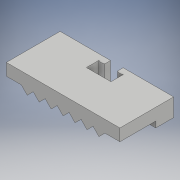
# Autodesk Inventor part: Clamp-part2(moving)-Base9x19mm.
Saved by Autodesk Inventor 2017 (Build 210142000, 142)
## iProperties
Created: 2021-08-04
Part Number: Clamp-part2(moving)-Base9x19mm.
Material: Generic
Document SubType Name: Modeling
Designer: Nikita
Density: 1 g/cm^3
Appearance: Default
Author: Nikita
Autodesk Inventor part; units mm, degrees
ref_plane "YZ Plane" through (0, 0, 0) normal (1, 0, 0) x (0, 1, 0)
ref_plane "XZ Plane" through (0, 0, 0) normal (0, 1, 0) x (-1, 0, 0)
ref_plane "XY Plane" through (0, 0, 0) normal (0, 0, 1) x (1, 0, 0)
sketch "Sketch1" plane through (0, 0, 0) normal (0, 0, 1) x (1, 0, 0)
  line L0 (0, 0) -> (19, 0)
  line L1 (19, 0) -> (19, 9)
  line L2 (19, 9) -> (0, 9)
  line L3 (0, 9) -> (0, 0)
  point P0 (9.5, 9)
  dimension "d0" = 19
  dimension "d1" = 9
  constraints: 8 end point, 2 parallel, 1 horizontal, 1 midpoint, 1 perpendicular
  measures "d0" distance of L2.end L1.end
  measures "d1" distance of L1.end L0.end
extrude "Extrusion1" add sketch "Sketch1" along normal blind 3
sketch "Sketch10" plane through (0, 0, 0) normal (-1, 0, 0) x (0, 0, 1)
  line L0 (0, 0) -> (3, 0) projected
  line L1 (3, 9) -> (3, 0) projected
  line L2 (3, 0) -> (2, 0)
  line L3 (2, 0) -> (2, 6)
  line L4 (2, 6) -> (3, 6)
  line L5 (3, 6) -> (3, 0)
  line L6 (3, 0) -> (2, 1)
  line L7 (3, 0) -> (4.4142, 0) construction
  line L8 (2, 1) -> (3, 2)
  line L9 (3, 0) -> (3, 9) projected
  line L10 (3, 2) -> (2, 3)
  line L11 (2, 3) -> (3, 4)
  line L12 (2, 5) -> (3, 4)
  line L13 (2, 5) -> (3, 5)
  dimension "d23" = 1
  dimension "d24" = 6
  dimension "d25" = 135
  dimension "d26" = 90
  constraints: 22 end point, 5 point on line, 3 perpendicular, 2 horizontal, 2 parallel, 1 equal length, 1 midpoint
  measures "d23" distance of L4.end L3.end
  measures "d24" distance of L2.end L3.end
  measures "d25" angle of L7 L6
  measures "d26" angle of L6 L8
extrude "Extrusion8" cut sketch "Sketch10" against normal up to next contours L6 L8 L1 | L10 L11 L1 | L12 L13 L1 | L3 L4 L1 L13
sketch "Sketch12" plane through (0, 0, 3) normal (0, 0, 1) x (1, 0, 0)
  line L0 (19, 9) -> (0, 9) projected
  line L1 (11.5494, 5.95) -> (7.4494, 5.95)
  line L2 (7.4494, 5.95) -> (7.4494, 8.05)
  line L3 (7.4494, 8.05) -> (11.5494, 8.05)
  line L4 (11.5494, 8.05) -> (11.5494, 5.95)
  line L5 (11.5494, 5.95) -> (7.4494, 8.05) construction
  line L6 (7.4494, 5.95) -> (11.5494, 8.05) construction
  line L7 (10.5494, 7.1) -> (8.4494, 7.1)
  line L8 (8.4494, 7.1) -> (8.4494, 9)
  line L9 (8.4494, 9) -> (10.5494, 9)
  line L10 (10.5494, 9) -> (10.5494, 7.1)
  line L11 (10.5494, 7.1) -> (8.4494, 9) construction
  line L12 (8.4494, 7.1) -> (10.5494, 9) construction
  point P0 (0, 0)
  point P1 (9.4994, 7)
  point P2 (9.4994, 8.05)
  dimension "d47" = 2
  dimension "d48" = 4.1
  dimension "d49" = 2.1
  dimension "d50" = 2.1
  constraints: 24 end point, 5 midpoint, 4 parallel, 2 horizontal, 2 perpendicular, 1 point on line
  measures "d47" distance from line of L0 point (9.499, 7)
  measures "d48" distance of L2.end L3.end
  measures "d49" distance of L1.end L2.end
  measures "d50" distance of L8.end L9.end
extrude "Extrusion10" cut sketch "Sketch12" against normal up to next
sketch "Sketch14" plane through (0, 0, 2) normal (0, 0, 1) x (1, 0, 0)
  line L0 (6.4994, 5) -> (12.4994, 5)
  line L1 (12.4994, 5) -> (12.4994, 6)
  line L2 (12.4994, 6) -> (6.4994, 6)
  line L3 (6.4994, 6) -> (6.4994, 5)
  line L4 (6.4994, 5) -> (12.4994, 6) construction
  line L5 (12.4994, 5) -> (6.4994, 6) construction
  line L6 (19, 9) -> (10.5494, 9) projected
  point P0 (0, 0)
  point P1 (9.4994, 5.5)
  dimension "d57" = 6
  dimension "d58" = 1
  dimension "d59" = 3.5
  constraints: 12 end point, 2 midpoint, 2 parallel, 1 horizontal, 1 perpendicular
  measures "d57" distance of L2.end L1.end
  measures "d58" distance of L1.end L0.end
  measures "d59" distance from line of L6 point (9.499, 5.5)
extrude "Extrusion12" add sketch "Sketch14" along normal blind 1
chamfer "Chamfer1" distance 0.5 angle 45 1 edges at (9.4994, 5, 3)
sketch "Sketch16" plane through (0, 0, 0) normal (0, 0, -1) x (-1, 0, 0)
  line L0 (-11.5494, 8.05) -> (-11.5494, 6) projected
  line L1 (-10.5494, 8.05) -> (-11.5494, 8.05) projected
  arc A0 (-11.5494, 8.05) -> (-10.5494, 8.05) centre (-11.0494, 8.916) ccw
  line L2 (-8.4494, 8.05) -> (-7.4494, 8.05) projected
  arc A1 (-8.4494, 8.05) -> (-7.4494, 8.05) centre (-7.9494, 8.916) ccw
  point P0 (0, 0)
  dimension "d66" = 1
  dimension "d67" = 1
  constraints: 4 point on circle, 2 centre point
  measures "d66" radius of A0
  measures "d67" radius of A1
extrude "Extrusion13" add sketch "Sketch16" against normal up to surface (3 mm away)
sketch "Sketch18" plane through (0, 0, 0) normal (0, -1, 0) x (1, 0, 0)
  line L0 (9.5, 3) -> (8.5, 2)
  line L1 (9.5, 3) -> (10.9142, 3) construction
  line L2 (8.5, 2) -> (7.5, 3)
  line L3 (7.5, 3) -> (6.4994, 2)
  line L4 (6.4994, 2) -> (5.5, 3)
  line L5 (5.5, 3) -> (4.5, 2)
  line L6 (5.5, 3) -> (6.9142, 3) construction
  line L7 (4.5, 2) -> (3.5, 3)
  line L8 (3.5, 3) -> (2.5, 2)
  line L9 (0, 3) -> (6.4994, 3) projected
  line L10 (0, 3) -> (3.5, 3)
  line L11 (19, 3) -> (19, 2)
  line L12 (19, 2) -> (16.5, 2)
  line L13 (0, 2) -> (0, 3)
  line L14 (8.5, 2) -> (6.4994, 2)
  line L15 (6.4994, 2) -> (4.5, 2)
  line L16 (4.5, 2) -> (2.5, 2)
  line L17 (3.5, 3) -> (5.5, 3)
  line L18 (5.5, 3) -> (7.5, 3)
  line L19 (7.5, 3) -> (9.5, 3)
  line L20 (2.5, 2) -> (0, 2)
  line L21 (9.5, 2.2481) -> (9.5, 2.7918)
  line L22 (9.5, 3) -> (10.5, 2)
  line L23 (10.5, 2) -> (11.5, 3)
  line L24 (11.5, 3) -> (12.5006, 2)
  line L25 (12.5006, 2) -> (13.5, 3)
  line L26 (13.5, 3) -> (14.5, 2)
  line L27 (14.5, 2) -> (15.5, 3)
  line L28 (15.5, 3) -> (16.5, 2)
  line L29 (14.5, 2) -> (12.5006, 2)
  line L30 (16.5, 2) -> (14.5, 2)
  line L31 (12.5006, 2) -> (10.5, 2)
  line L32 (10.5, 2) -> (8.5, 2)
  line L33 (11.5, 3) -> (13.5, 3)
  line L34 (13.5, 3) -> (15.5, 3)
  line L35 (15.5, 3) -> (19, 3)
  line L36 (9.5, 3) -> (11.5, 3)
  point P0 (0, 0)
  dimension "d71" = 135
  dimension "d72" = 90
  dimension "d73" = 135
  constraints: 73 parallel, 72 end point, 11 perpendicular, 10 horizontal, 7 symmetric about line, 2 equal length, 1 vertical
  measures "d71" angle of L0 L1
  measures "d72" angle of L0 L2
  measures "d73" angle of L5 L6
extrude "Extrusion14" cut sketch "Sketch18" against normal blind 5 contours L0 L2 L19 | L36 L23 L22 | L3 L4 L9 L18 | L33 L25 L24 | L34 L27 L26 | L5 L7 L9 | L35 L11 L12 L28 | L8 L20 L13 L9
body "Solid1"
